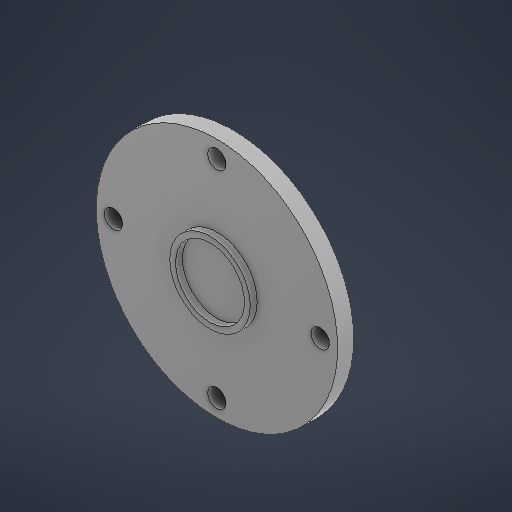
# Autodesk Inventor part: Diff_Driveshaft_Output_V1
Saved by Autodesk Inventor 2026.1 (Build 301233000, 233)
## iProperties
Created: 2026-08-05
Part Number: Diff_Driveshaft_Output_V1
Material: Generic
Document SubType Name: Modeling
Designer: share
Density: 1 g/cm^3
Appearance: Default
Author: share
Autodesk Inventor part; units mm, degrees
ref_plane "YZ Plane" through (0, 0, 0) normal (1, 0, 0) x (0, 1, 0)
ref_plane "XZ Plane" through (0, 0, 0) normal (0, 1, 0) x (-1, 0, 0)
ref_plane "XY Plane" through (0, 0, 0) normal (0, 0, 1) x (1, 0, 0)
sketch "Sketch1" plane through (0, 0, 0) normal (0, 0, 1) x (1, 0, 0)
  circle A0 centre (0, 0) radius 52.5
  dimension "d0" = 105
  constraints: 1 centre point, 1 coincident
  measures "d0" diameter of A0
extrude "Extrusion1" add sketch "Sketch1" against normal blind 7
sketch "Sketch2" plane through (0, 0, 0) normal (0, 0, 1) x (1, 0, 0)
  circle A0 centre (0, 0) radius 45 construction
  line L0 (0, 0) -> (0, 45) construction
  dimension "d3" = 90
  constraints: 2 coincident, 2 end point, 1 vertical, 1 vertical alignment, 2 other
hole "Hole1" at (0, 45, 0) direction (0, 0, -1) diameter 8 depth 7
pattern_circular "Circular Pattern1" count 4 over 360 about axis through (0, 0, -10) along (0, 0, 1) of "Hole1"
sketch "Sketch3" plane through (0, 0, -7) normal (0, 0, -1) x (-1, 0, 0)
  circle A0 centre (0, 0) radius 10
  dimension "d14" = 20
  constraints: 1 centre point, 1 coincident
  measures "d14" diameter of A0
extrude "Extrusion2" add sketch "Sketch3" along normal blind 30
sketch "Sketch4" plane through (0, 0, 0) normal (0, 0, 1) x (1, 0, 0)
  circle A0 centre (0, 0) radius 15
  circle A1 centre (0, 0) radius 17.5
  dimension "d17" = 35
  dimension "d18" = 30
  constraints: 2 centre point, 2 coincident
  measures "d17" diameter of A1
  measures "d18" diameter of A0
extrude "Extrusion3" add sketch "Sketch4" along normal blind 3
body "Solid1"
